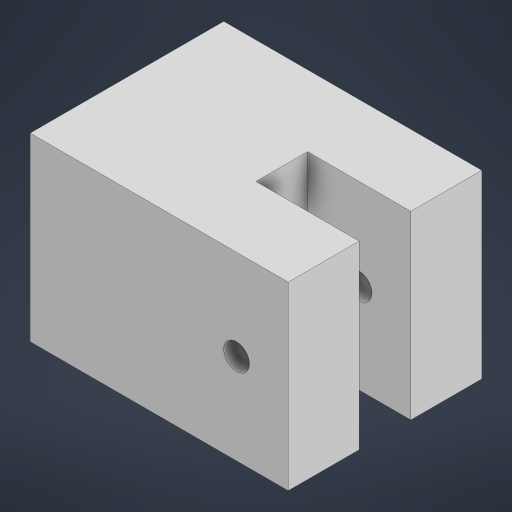
# Autodesk Inventor part: Slider
Saved by Autodesk Inventor 2024 (Build 280153000, 153)
## iProperties
Created: 2023-12-06
Part Number: Slider
Material: Generic
Document SubType Name: Modeling
Designer: calvi
Density: 1 g/cm^3
Appearance: Default
Author: calvi
Autodesk Inventor part; units mm, degrees
ref_plane "YZ Plane" through (0, 0, 0) normal (1, 0, 0) x (0, 1, 0)
ref_plane "XZ Plane" through (0, 0, 0) normal (0, 1, 0) x (-1, 0, 0)
ref_plane "XY Plane" through (0, 0, 0) normal (0, 0, 1) x (1, 0, 0)
sketch "Sketch1" plane through (0, 0, 0) normal (0, 0, 1) x (1, 0, 0)
  line L0 (0, 0) -> (50.8, 0)
  line L1 (50.8, 0) -> (50.8, 35.56)
  line L2 (50.8, 35.56) -> (0, 35.56)
  line L3 (0, 35.56) -> (0, 0)
  dimension "d0" = 50.8
  dimension "d1" = 35.56
  constraints: 8 end point, 2 parallel, 1 horizontal, 1 perpendicular
  measures "d0" distance of L2.end L1.end
  measures "d1" distance of L1.end L0.end
extrude "Extrusion1" add sketch "Sketch1" along normal blind 38.1
sketch "Sketch2" plane through (0, 35.56, 0) normal (0, 1, 0) x (1, 0, 0)
  line L0 (50.8, 0) -> (50.8, -38.1) projected
  line L1 (50.8, -13.97) -> (25.4, -13.97)
  line L2 (25.4, -13.97) -> (25.4, -24.13)
  line L3 (25.4, -24.13) -> (50.8, -24.13)
  line L4 (50.8, -24.13) -> (50.8, -13.97)
  line L5 (50.8, -38.1) -> (0, -38.1) projected
  point P0 (0, 0)
  dimension "d4" = 25.4
  dimension "d5" = 10.16
  dimension "d6" = 13.97
  constraints: 8 end point, 2 parallel, 1 horizontal, 1 perpendicular, 1 point on line
  measures "d4" distance of L3.end L2.end
  measures "d5" distance of L2.end L1.end
  measures "d6" distance between parallel lines of L5 L3
extrude "Extrusion2" cut sketch "Sketch2" against normal blind 57.15
sketch "Sketch3" plane through (50.8, 35.56, 24.13) normal (0, 0, -1) x (-1, 0, 0)
  circle A0 centre (10.16, -17.78) radius 2.54
  line L0 (25.4, -35.56) -> (0, -35.56) projected
  line L1 (0, -35.56) -> (0, 0) projected
  point P0 (50.8, -35.56)
  dimension "d9" = 5.08
  dimension "d10" = 17.78
  dimension "d11" = 10.16
  constraints: 1 centre point
  measures "d9" diameter of A0
  measures "d10" distance from line of L0 A0.centre
  measures "d11" distance from line of L1 A0.centre
extrude "Extrusion3" cut sketch "Sketch3" against normal blind 57.15
sketch "Sketch4" plane through (50.8, 35.56, 24.13) normal (0, 0, -1) x (-1, 0, 0)
  circle A0 centre (10.16, -17.78) radius 2.54 projected
  circle A1 centre (10.16, -17.78) radius 2.54
  point P0 (50.8, -35.56)
  constraints: 1 centre point, 1 coincident
extrude "Extrusion4" cut sketch "Sketch4" along normal blind 57.15
sketch "Sketch5" plane through (25.4, 35.56, 24.13) normal (1, 0, 0) x (0, 0, -1)
  line L0 (0, 0) -> (0, -35.56) projected
  line L1 (10.16, -35.56) -> (0, -35.56) projected
  line L2 (0, 0) -> (10.16, 0)
  line L3 (10.16, 0) -> (10.16, -35.56)
  line L4 (10.16, -35.56) -> (0, -35.56)
  line L5 (0, -35.56) -> (0, 0)
  point P0 (24.13, -35.56)
  constraints: 8 end point, 2 parallel, 1 horizontal, 1 perpendicular
extrude "Extrusion5" add sketch "Sketch5" along normal blind 5.08
sketch "Sketch6" plane through (0, 0, 38.1) normal (0, 0, 1) x (1, 0, 0)
  line L0 (30.48, 0) -> (30.48, 35.56) projected
  line L1 (30.48, 35.56) -> (30.48, 0)
  line L2 (0, 35.56) -> (30.48, 35.56)
  arc A0 (30.48, 0) -> (30.48, 35.56) centre (30.48, 17.78) ccw
  point P0 (0, 0)
  constraints: 4 end point, 2 point on circle, 1 centre point, 1 collinear, 1 perpendicular, 1 tangent
body "Solid1"
